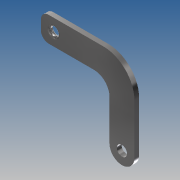
# Autodesk Inventor part: DD_KVD_002_10
Saved by Autodesk Inventor 2017.3 (Build 213256000, 256)
## iProperties
Created: 2023-11-02
Part Number: DD_KVD_002_10
Material: Nerezová ocel
Document SubType Name: Sheet Metal
Designer: Darena
Density: 8 g/cm^3
Sheet Metal Rule: Výchozí_mm
Appearance: Pololeštěná
Flat Pattern Width: 12 cm
Flat Pattern Length: 12 cm
Flat Pattern Area: 144 cm^2
Sheet Metal Width: 120,000 mm
Sheet Metal Length: 120,000 mm
Sheet Metal Area: 14400,000 mm^2
Author: Darena
Autodesk Inventor part; units mm, degrees
ref_plane "YZ Plane" through (0, 0, 0) normal (1, 0, 0) x (0, 1, 0)
ref_plane "XZ Plane" through (0, 0, 0) normal (0, 1, 0) x (-1, 0, 0)
ref_plane "XY Plane" through (0, 0, 0) normal (0, 0, 1) x (1, 0, 0)
sketch "Náčrt2" plane through (0, 0, 0) normal (0, 1, 0) x (-1, 0, 0)
  line L0 (11.5, 17.5) -> (-11.5, 17.5) construction
  line L1 (-17.5, 11.5) -> (-17.5, -11.5) construction
  line L2 (-11.5, -17.5) -> (11.5, -17.5) construction
  line L3 (17.5, -11.5) -> (17.5, 11.5) construction
  line L4 (42.5, 36) -> (42.5, -77.5) construction
  line L5 (9, -22.5) -> (-14, -22.5) construction
  line L6 (-20, -28.5) -> (-20, -51.5) construction
  line L7 (-14, -57.5) -> (9, -57.5) construction
  line L8 (15, -51.5) -> (15, -28.5) construction
  arc A0 (15, -28.5) -> (9, -22.5) centre (9, -28.5) ccw construction
  arc A1 (9, -57.5) -> (15, -51.5) centre (9, -51.5) ccw construction
  arc A2 (-20, -51.5) -> (-14, -57.5) centre (-14, -51.5) ccw construction
  arc A3 (-14, -22.5) -> (-20, -28.5) centre (-14, -28.5) ccw construction
  line L9 (-45.6938, -20) -> (9, -20) construction
  arc A4 (17.5, -28.5) -> (9, -20) centre (9, -28.5) ccw construction
  line L10 (17.5, -28.5) -> (17.5, -51.5) construction
  line L11 (17.5, -51.5) -> (15, -51.5) construction
  line L12 (-14, -22.5) -> (-45.6938, -22.5) construction
  line L13 (-45.6938, -22.5) -> (-45.6938, -20) construction
  arc A5 (17.5, 11.5) -> (11.5, 17.5) centre (11.5, 11.5) ccw construction
  arc A6 (11.5, -17.5) -> (17.5, -11.5) centre (11.5, -11.5) ccw construction
  arc A7 (-17.5, -11.5) -> (-11.5, -17.5) centre (-11.5, -11.5) ccw construction
  arc A8 (-11.5, 17.5) -> (-17.5, 11.5) centre (-11.5, 11.5) ccw construction
  line L14 (-11.5, -20) -> (11.5, -20) construction
  line L15 (-20, 73.4113) -> (-20, -11.5) construction
  arc A9 (-20, -11.5) -> (-11.5, -20) centre (-11.5, -11.5) ccw construction
  line L16 (-17.5, 11.5) -> (-17.5, 73.4113) construction
  line L17 (-17.5, 73.4113) -> (-20, 73.4113) construction
  line L18 (11.5, -20) -> (11.5, -17.5) construction
  line L19 (17.5, 17.5) -> (-17.5, 17.5) construction
  line L20 (-17.5, 17.5) -> (-17.5, 52.5) construction
  line L21 (-17.5, 52.5) -> (17.5, 52.5) construction
  line L22 (17.5, 52.5) -> (17.5, 17.5) construction
  circle A10 centre (0, 35) radius 6.5
  arc A11 (0, 51) -> (0, 19) centre (0, 35) ccw construction
  line L23 (0, 51) -> (27.5, 51) construction
  line L24 (0, 19) -> (11.5, 19) construction
  line L25 (27.5, 51) -> (42.5, 36) construction
  arc A12 (17.5, 13) -> (11.5, 19) centre (11.5, 13) ccw construction
  line L26 (17.5, 13) -> (17.5, -51.5) construction
  line L27 (-13.5, -57.5) -> (-13.5, -59.2574) construction
  line L28 (-12.6213, -61.3787) -> (14.1066, -88.1066) construction
  line L29 (24.7132, -92.5) -> (27.5, -92.5) construction
  arc A13 (27.5, -92.5) -> (42.5, -77.5) centre (27.5, -77.5) ccw construction
  arc A14 (14.1066, -88.1066) -> (24.7132, -92.5) centre (24.7132, -77.5) ccw construction
  arc A15 (-13.5, -59.2574) -> (-12.6213, -61.3787) centre (-10.5, -59.2574) ccw construction
  line L30 (17.5, -51.5) -> (17.5, -51.5) construction
  line L31 (6.4677, -58.2408) -> (-10.5, -57.5) construction
  line L32 (-13.5, -57.5) -> (-10.5, -57.5) construction
  line L33 (6.4677, -58.2408) -> (6.5, -57.5) construction
  line L34 (6.5, -57.5) -> (11.5, -57.5) construction
  arc A16 (11.5, -57.5) -> (17.5, -51.5) centre (11.5, -51.5) ccw construction
  arc A17 (-16, 35) -> (16, 35) centre (0, 35) ccw
  line L35 (16, 35) -> (16, 87)
  line L36 (-16, 35) -> (-16, 99)
  line L37 (24, 139) -> (94, 139)
  line L38 (104, 129) -> (104, 117)
  line L39 (94, 107) -> (36, 107)
  arc A18 (36, 107) -> (16, 87) centre (36, 87) ccw
  arc A19 (24, 139) -> (-16, 99) centre (24, 99) ccw
  arc A20 (104, 129) -> (94, 139) centre (94, 129) ccw
  arc A21 (94, 107) -> (104, 117) centre (94, 117) ccw
  point P0 (0, 0)
  point P1 (17.5, 0)
  point P2 (0, 17.5)
  point P3 (42.5, 51)
  point P4 (17.5, 35)
  point P5 (0, 52.5)
  point P6 (-13.5, -60.5)
  point P7 (16, 107)
  point P8 (-16, 139)
  point P9 (104, 139)
  point P10 (104, 107)
  dimension "d34" = 35
  dimension "d35" = 6
  dimension "d36" = 5
  dimension "d37" = 2.5
  dimension "d38" = 2.5
  dimension "d39" = 6
  dimension "d40" = 2.5
  dimension "d43" = 25
  dimension "d46" = 13
  dimension "d47" = 32
  dimension "d48" = 15
  dimension "d49" = 15
  dimension "d50" = 6
  dimension "d51" = 35
  dimension "d55" = 3
  dimension "d56" = 15
  dimension "d57" = 15
  dimension "d58" = 3
  dimension "d60" = 35
  dimension "d61" = 3
  dimension "d62" = 2.5
  dimension "d63" = 35
  dimension "d64" = 45
  dimension "d66" = 31
  dimension "d69" = 6
  dimension "d72" = 2.5
  dimension "d79" = 32
  dimension "d80" = 120
  dimension "d81" = 120
  dimension "d82" = 20
  dimension "d83" = 40
  dimension "d85" = 10
  constraints: 80 end point, 45 point on circle, 37 tangent, 22 centre point, 18 point on line, 12 perpendicular, 8 parallel, 7 equal radius, 6 horizontal, 5 collinear, 5 vertical, 4 midpoint, 2 coincident, 2 horizontal alignment, 2 vertical alignment, 3 other
  measures "d34" distance between parallel lines of L7 L5
  measures "d35" radius of A0
  measures "d36" distance between parallel lines of L2 L5
  measures "d37" distance between parallel lines of L1 L6
  measures "d38" distance between parallel lines of L5 L9
  measures "d39" radius of A5
  measures "d40" radial gap between concentric circles of A7 A9
  measures "d43" distance between parallel lines of L4 L10
  measures "d46" diameter of A10
  measures "d47" diameter of A11
  measures "d48" distance of L23.end point (42.5, 51)
  measures "d49" distance of L4.start point (42.5, 51)
  measures "d50" radius of A12
  measures "d51" distance between parallel lines of L0 L2
  measures "d55" distance of L27.start point (-13.5, -60.5)
  measures "d56" radius of A13
  measures "d57" radius of A14
  measures "d58" radius of A15
  measures "d60" distance between parallel lines of L1 L3
  measures "d61" distance of L27.start L31.end
  measures "d62" angle of L31 L7
  measures "d63" distance between parallel lines of L29 L7
  measures "d64" angle of L28 L7
  measures "d66" distance from line of L27.start L26
  measures "d69" radius of A16
  measures "d72" distance of L33.end L7.end
  measures "d79" distance between parallel lines of L37 L39
  measures "d80" distance from line of L24.start L37
  measures "d81" distance between parallel lines of L38 L36
  measures "d82" radius of A18
  measures "d83" radius of A19
  measures "d85" radius of A20
extrude "Vysunutí1" add sketch "Náčrt2" along normal blind 6
sketch "Náčrt5" plane through (0, 0, 0) normal (0, -1, 0) x (1, 0, 0)
  circle A0 centre (0, 35) radius 6.5 projected
  arc A1 (-16, 35) -> (16, 35) centre (0, 35) ccw projected
  line L0 (16, 99) -> (16, 35) projected
  line L1 (-16, 35) -> (-16, 87) projected
  circle A2 centre (-88, 123) radius 5
  arc A3 (16, 99) -> (-24, 139) centre (-24, 99) ccw projected
  line L2 (-94, 139) -> (-24, 139) projected
  line L3 (-104, 117) -> (-104, 129) projected
  line L4 (-36, 107) -> (-94, 107) projected
  arc A4 (-16, 87) -> (-36, 107) centre (-36, 87) ccw projected
  arc A5 (-94, 139) -> (-104, 129) centre (-94, 129) ccw projected
  arc A6 (-104, 117) -> (-94, 107) centre (-94, 117) ccw projected
  point P0 (0, 0)
  point P1 (-104, 123)
  dimension "d75" = 10
  dimension "d84" = 16
  constraints: 1 centre point, 1 horizontal alignment, 1 midpoint
  measures "d75" diameter of A2
  measures "d84" distance from line of A2.centre L3
extrude "Vysunutí3" cut sketch "Náčrt5" against normal blind 10 contours A2
fillet "Zaoblení6" radius 3 2 edges at (-93, 0, 123) (-93, 6, 123)
equation "\"d49\" = d48"
equation "\"d79\" = d47"
equation "\"d81\" = d80"
equation "\"PoloměrOhybu\" = Tloušťka"
equation "\"ŠířkaVýštipu\" = Tloušťka"
equation "\"HloubkaVýštipu\" = 0.5 * Tloušťka"
equation "\"VelikostRohovéhoVýštipu\" = 4 * Tloušťka"
equation "\"MinimálníZbytek\" = 2 * Tloušťka"
equation "\"PřechodovýPoloměr\" = PoloměrOhybu"
equation "\"VelikostJacobihoPoloměru\" = PoloměrOhybu"
equation "\"VelikostMezery\" = Tloušťka"
equation "\"Tloušťka\" = 6"
